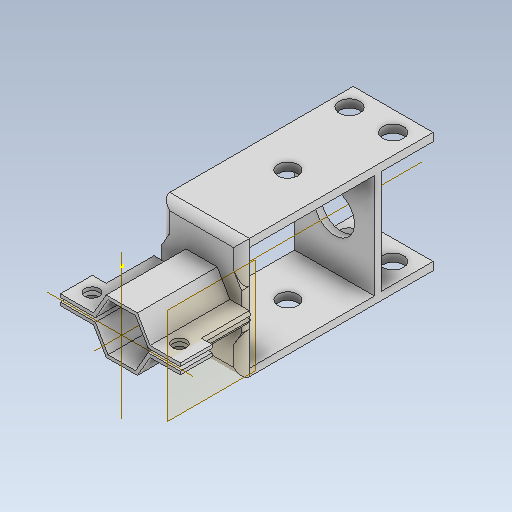
# Autodesk Inventor part: suction_cup_holder
Saved by Autodesk Inventor 2021 (Build 250183000, 183)
## iProperties
Created: 2023-04-09
Part Number: suction_cup_holder
Material: Generic
Document SubType Name: Modeling
Designer: mahmo
Density: 1 g/cm^3
Appearance: Default
Author: mahmo
Autodesk Inventor part; units mm, degrees
ref_plane "XZ Plane" through (0, 0, 0) normal (0, 1, 0) x (-1, 0, 0)
ref_plane "XY Plane" through (0, 0, 0) normal (0, 0, 1) x (1, 0, 0)
sketch "Sketch1" plane through (0, 0, 0) normal (0, 0, 1) x (1, 0, 0)
  line L0 (3.45, -5.9756) -> (-3.45, -5.9756)
  line L1 (-3.45, -5.9756) -> (-6.9, 0)
  line L2 (-6.9, 0) -> (-3.45, 5.9756)
  line L3 (-3.45, 5.9756) -> (3.45, 5.9756)
  line L4 (3.45, 5.9756) -> (6.9, 0)
  line L5 (6.9, 0) -> (3.45, -5.9756)
  line L6 (0, 0) -> (10.8127, 0) construction
  line L7 (6.3368, 10.9756) -> (-6.3368, 10.9756)
  line L8 (-6.3368, 10.9756) -> (-12.6735, 0)
  line L9 (-12.6735, 0) -> (-6.3368, -10.9756)
  line L10 (-6.3368, -10.9756) -> (6.3368, -10.9756)
  line L11 (6.3368, -10.9756) -> (12.6735, 0)
  line L12 (12.6735, 0) -> (6.3368, 10.9756)
  dimension "d0" = 6.9
  dimension "d1" = 5
  constraints: 26 end point, 1 coincident, 1 horizontal, 1 parallel, 18 other
  measures "d0" distance of L2.end L3.end
  measures "d1" distance between parallel lines of L3 L7
extrude "Extrusion1" add sketch "Sketch1" against normal blind 20 contours L0 L1 L2 L3 L4 L5 | L12 L11 L10 L9 L8 L7
sketch "Sketch4" plane through (0, 0, 0) normal (0, 0, 1) x (1, 0, 0)
  line L0 (6.9, 0) -> (3.45, -5.9756)
  line L1 (3.45, -5.9756) -> (-3.45, -5.9756)
  line L2 (-3.45, -5.9756) -> (-6.9, 0)
  line L3 (-6.9, 0) -> (-3.45, 5.9756)
  line L4 (-3.45, 5.9756) -> (3.45, 5.9756)
  line L5 (3.45, 5.9756) -> (6.9, 0)
  point P0 (0, 0)
  point P1 (0, 0)
  dimension "d7" = 6.9
  constraints: 12 end point, 1 coincident, 13 other
  measures "d7" distance of L3.end L4.end
extrude "Extrusion3" cut sketch "Sketch4" against normal blind 10
sketch "Sketch5" plane through (0, 0, -10) normal (0, 0, 1) x (1, 0, 0)
  circle A0 centre (0, 0) radius 5
  dimension "d10" = 10
  constraints: 1 centre point, 1 coincident
  measures "d10" diameter of A0
extrude "Extrusion4" cut sketch "Sketch5" against normal blind 10
sketch "Sketch6" plane through (0, 0, 0) normal (0, 0, 1) x (1, 0, 0)
  line L0 (-12.8409, -0.5) -> (12.8409, -0.5)
  line L1 (12.8409, -0.5) -> (12.8409, 0.5)
  line L2 (12.8409, 0.5) -> (-12.8409, 0.5)
  line L3 (-12.8409, 0.5) -> (-12.8409, -0.5)
  line L4 (-12.8409, -0.5) -> (12.8409, 0.5) construction
  line L5 (12.8409, -0.5) -> (-12.8409, 0.5) construction
  point P0 (0, 0)
  dimension "d13" = 1
  constraints: 12 end point, 2 midpoint, 2 parallel, 1 horizontal, 1 perpendicular
  measures "d13" distance of L1.end L0.end
extrude "Extrusion5" cut sketch "Sketch6" against normal blind 10
ref_plane "Work Plane1" through (12.3848, 0.5, 0) normal (1, 0, 0) x (0, 1, 0)
sketch "Sketch7" plane through (12.3848, 0.5, 0) normal (1, 0, 0) x (0, 1, 0)
  line L0 (0, -10) -> (0, 0) projected
  line L1 (0, 0) -> (0.8, 0)
  line L2 (0.8, 0) -> (0.8, -8)
  line L3 (0.8, -8) -> (0, -8)
  line L4 (0, -8) -> (0, 0)
  point P0 (-0.5, 0)
  point P1 (0, -8)
  dimension "d16" = 0.8
  dimension "d17" = 8
  constraints: 8 end point, 2 parallel, 1 horizontal, 1 perpendicular
  measures "d16" distance of L2.end L3.end
  measures "d17" distance of L1.end L2.end
extrude "Extrusion6" add sketch "Sketch7" along normal blind 8 and the other way blind 1
mirror "Mirror1" about plane through (0, 0, 0) normal (0, 1, 0) of "Extrusion6"
mirror "Mirror2" about plane through (0, 0, 0) normal (1, 0, 0) of "Extrusion6", "Mirror1"
sketch "Sketch8" plane through (11.9229, 1.3, 0) normal (0, 1, 0) x (1, 0, 0)
  circle A0 centre (4.7784, 4.2209) radius 1.75
  point P0 (-11.9229, 0)
  dimension "d22" = 3.5
  constraints: 1 centre point
  measures "d22" diameter of A0
extrude "Extrusion7" cut sketch "Sketch8" against normal blind 5
mirror "Mirror3" about plane through (0, 0, 0) normal (1, 0, 0) of "Extrusion7"
sketch "Sketch9" plane through (0, 0, -20) normal (0, 0, -1) x (-1, 0, 0)
  line L0 (-10, 15) -> (10, 15)
  line L1 (10, 15) -> (10, -15)
  line L2 (10, -15) -> (-10, -15)
  line L3 (-10, -15) -> (-10, 15)
  line L4 (-10, 15) -> (10, -15) construction
  line L5 (10, 15) -> (-10, -15) construction
  circle A0 centre (0, 0) radius 5 projected
  dimension "d25" = 20
  dimension "d26" = 30
  constraints: 12 end point, 2 midpoint, 2 parallel, 1 horizontal, 1 perpendicular
  measures "d25" distance of L1.end L2.end
  measures "d26" distance of L0.end L1.end
extrude "Extrusion8" add sketch "Sketch9" along normal blind 35
fillet "Fillet1" radius 2 6 edges at (-10, 9.8153, -20) (0, 15, -20) (10, 9.8153, -20) (-10, -9.8153, -20) (10, -9.8153, -20) (0, -15, -20)
sketch "Sketch10" plane through (-10, 15, -55) normal (0, 1, 0) x (1, 0, 0)
  circle A0 centre (10, -13.383) radius 2.5
  point P0 (10, -55)
  dimension "d30" = 5
  constraints: 1 centre point
  measures "d30" diameter of A0
extrude "Extrusion9" cut sketch "Sketch10" against normal blind 35
sketch "Sketch11" plane through (0, 0, -55) normal (0, 0, -1) x (-1, 0, 0)
  line L0 (10, 15) -> (-10, 15) projected
  line L1 (10, -15) -> (10, 15) projected
  line L2 (-10, 15) -> (10, 15)
  line L3 (10, 15) -> (10, 12)
  line L4 (10, 12) -> (-10, 12)
  line L5 (-10, 12) -> (-10, 15)
  line L6 (-10, 15) -> (-10, -15) projected
  line L7 (10, -15) -> (-10, -15)
  line L8 (-10, -15) -> (-10, -12)
  line L9 (-10, -12) -> (10, -12)
  line L10 (10, -12) -> (10, -15)
  point P0 (0, 0)
  dimension "d33" = 3
  dimension "d34" = 3
  constraints: 16 end point, 4 parallel, 2 horizontal, 2 perpendicular, 2 point on line
  measures "d33" distance of L2.end L3.end
  measures "d34" distance of L7.end L8.end
extrude "Extrusion10" add sketch "Sketch11" along normal blind 10 contours L1 L4 L5 L0 | L1 L7 L6 L9
sketch "Sketch12" plane through (-10, 15, -22) normal (0, 1, 0) x (1, 0, 0)
  point P0 (10, -22)
sketch "Sketch14" plane through (-10, 15, -22) normal (0, 1, 0) x (1, 0, 0)
  point P0 (10, -22)
sketch "Sketch16" plane through (-10, -15, -22) normal (0, -1, 0) x (1, 0, 0)
  circle A0 centre (15, -41) radius 1.6 projected
  circle A1 centre (4.0698, -41) radius 1.6 projected
  point P0 (10, 22)
extrude "Extrusion13" cut sketch "Sketch16" against normal blind 33
sketch "Sketch17" plane through (0, 0, -65) normal (0, 0, -1) x (-1, 0, 0)
  line L0 (8, 13) -> (-8, 13) projected
  line L1 (-10, 12) -> (10, 12) projected
  line L2 (10, 12) -> (10, 15) projected
  line L3 (10, 15) -> (-10, 15) projected
  line L4 (-10, 15) -> (-10, 12) projected
  line L5 (10, -15) -> (10, -12) projected
  line L6 (10, -12) -> (-10, -12) projected
  line L7 (-10, -12) -> (-10, -15) projected
  line L8 (-10, -15) -> (10, -15) projected
  point P0 (0, 0)
extrude "Extrusion14" add sketch "Sketch17" along normal blind 3
sketch "Sketch18" plane through (0, 0, 0) normal (0, 0, 1) x (1, 0, 0)
  line L0 (-6.6113, 0.5) -> (-20.3848, 0.5) projected
  line L1 (-6.6113, 0.5) -> (-3.45, 5.9756) projected
  line L2 (-3.45, 5.9756) -> (3.45, 5.9756) projected
  line L3 (3.45, 5.9756) -> (6.6113, 0.5) projected
  line L4 (6.6113, 0.5) -> (20.3848, 0.5) projected
  line L5 (20.3848, 1.3) -> (20.3848, 0.5) projected
  line L6 (20.3848, 1.3) -> (11.9229, 1.3) projected
  line L7 (11.9229, 1.3) -> (6.3368, 10.9756) projected
  line L8 (6.3368, 10.9756) -> (-6.3368, 10.9756) projected
  line L9 (-6.3368, 10.9756) -> (-11.9229, 1.3) projected
  line L10 (-20.3848, 1.3) -> (-11.9229, 1.3) projected
  line L11 (-20.3848, 1.3) -> (-20.3848, 0.5) projected
  line L12 (-11.9229, 1.3) -> (-9.4981, 1.3)
  line L13 (-3.9119, 6.7756) -> (-7.0732, 1.3)
  line L14 (-7.0732, 1.3) -> (-10.9992, 1.3)
  line L15 (-10.9992, 1.3) -> (-5.8749, 10.1756)
  line L16 (-5.8749, 10.1756) -> (5.8749, 10.1756)
  line L17 (5.8749, 10.1756) -> (10.9992, 1.3)
  line L18 (10.9992, 1.3) -> (7.0732, 1.3)
  line L19 (7.0732, 1.3) -> (3.9119, 6.7756)
  line L20 (3.9119, 6.7756) -> (-3.9119, 6.7756)
  line L21 (10.9992, 1.3) -> (11.9229, 1.3)
  point P0 (0, 0)
  constraints: 20 end point, 2 horizontal, 7 other
extrude "Extrusion15" cut sketch "Sketch18" against normal blind 20 contours L9 L8 L7 L21 L17 L16 L15 L12 | L15 L16 L17 L18 L19 L20 L13 L14 L12
mirror "Mirror4" about plane through (0, 0, 0) normal (0, 1, 0) of "Extrusion15"
sketch "Sketch19" plane through (11.9229, 1.3, -8) normal (0, 1, 0) x (1, 0, 0)
  circle A0 centre (-1.5413, -3.9241) radius 1.75
  point P0 (-11.9229, -8)
  dimension "d49" = 3.5
  constraints: 1 centre point
  measures "d49" diameter of A0
extrude "Extrusion16" cut sketch "Sketch19" against normal blind 10
sketch "Sketch20" plane through (10, -1.3, -20) normal (1, 0, 0) x (0, 0, -1)
  line L0 (2, -13.7) -> (2, -3.3306) projected
  line L1 (33.3107, 13.3) -> (2, 13.3)
  line L2 (2, 13.3) -> (2, -10.8513)
  line L3 (2, -10.8513) -> (33.3107, -10.8513)
  line L4 (33.3107, -10.8513) -> (33.3107, 13.3)
  point P0 (-20, 1.3)
  constraints: 8 end point, 2 parallel, 1 horizontal, 1 perpendicular, 1 point on line
extrude "Extrusion17" cut sketch "Sketch20" against normal through all
sketch "Sketch21" plane through (0, 0, -10) normal (0, 0, 1) x (1, 0, 0)
  circle A0 centre (0, 0) radius 5 projected
  line L0 (-12.3848, 0.5) -> (-6.6113, 0.5) projected
  line L1 (-12.6735, 0) -> (-12.3848, 0.5) projected
  line L2 (-12.3848, -0.5) -> (-12.6735, 0) projected
  line L3 (-6.6113, -0.5) -> (-12.3848, -0.5) projected
  line L4 (-3.45, -5.9756) -> (-6.6113, -0.5) projected
  line L5 (3.45, -5.9756) -> (-3.45, -5.9756) projected
  line L6 (6.6113, -0.5) -> (3.45, -5.9756) projected
  line L7 (12.3848, -0.5) -> (6.6113, -0.5) projected
  line L8 (12.6735, 0) -> (12.3848, -0.5) projected
  line L9 (12.3848, 0.5) -> (12.6735, 0) projected
  line L10 (6.6113, 0.5) -> (12.3848, 0.5) projected
  line L11 (3.45, 5.9756) -> (6.6113, 0.5) projected
  line L12 (-3.45, 5.9756) -> (3.45, 5.9756) projected
  line L13 (-6.6113, 0.5) -> (-3.45, 5.9756) projected
  line L14 (6.6113, -0.5) -> (3.45, -5.9756) projected
  line L15 (6.6113, 0.5) -> (6.6113, -0.5)
  constraints: 2 end point, 1 vertical
extrude "Extrusion18" cut sketch "Sketch21" against normal up to surface (10 mm away) contours L10 L9 L8 L7 L15
mirror "Mirror5" about plane through (0, 0, 0) normal (1, 0, 0) of "Extrusion18"
move faces "Move1" translate (0, 1, 0) faces at (7.5, 15, -43.8723)
move faces "Move2" translate (0, 1, 0) faces at (0.1004, 12, -27.7117) (1.4775, 12, -57.168)
move faces "Move3" translate (0, -1, 0) faces at (1.4775, -12, -57.168) (0.1004, -12.1513, -27.7117)
move faces "Move4" translate (0, -1, 0) faces at (7.5, 16, -43.8723)
offset faces "Size1" outward -1 faces at (-4.9353, 0.8021, -21.3333) (4.9353, 0.8021, -13.3333)
move faces "Move5" translate (-5.75, 0, 0) faces at (20.3848, 0.7667, -5.3333) (20.3848, -0.7667, -5.3333)
move faces "Move6" translate (5, 0, 0) faces at (-20.3848, 0.7667, -5.3333) (-20.3848, -0.7667, -5.3333) (-18.4287, 1.0333, -3.9402) (-18.4287, -1.0333, -4.5017)
offset faces "Size2" outward -1 faces at (6.472, 14.3333, -62.3729) (-4.4582, 14.3333, -63.6271) (6.472, -13.6667, -62.3729) (-4.4582, -13.6667, -63.6271)
body "Solid1"
